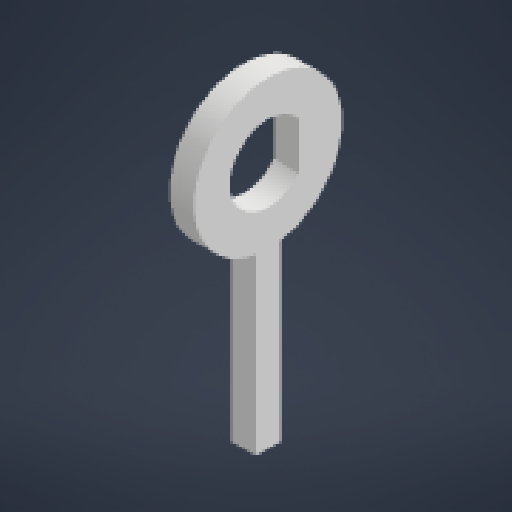
# Autodesk Inventor part: tarcza krańcówek
Saved by Autodesk Inventor 2026.1 (Build 301233020, 233B)
## iProperties
Created: 2026-03-17
Part Number: tarcza krańcówek
Material: Generic
Document SubType Name: Modeling
Designer: Jan
Density: 1 g/cm^3
Appearance: Default
Author: Jan
Autodesk Inventor part; units mm, degrees
ref_plane "YZ Plane" through (0, 0, 0) normal (1, 0, 0) x (0, 1, 0)
ref_plane "XZ Plane" through (0, 0, 0) normal (0, 1, 0) x (-1, 0, 0)
ref_plane "XY Plane" through (0, 0, 0) normal (0, 0, 1) x (1, 0, 0)
sketch "Sketch1" plane through (0, 0, 0) normal (1, 0, 0) x (0, 1, 0)
  arc A0 (1.9313, -2.4249) -> (-1.9054, -2.4453) centre (0, 0) ccw
  circle A1 centre (0, 0) radius 6
  line L0 (-3.1, 0) -> (-3.1, 2) construction
  line L1 (-1.9054, -2.4453) -> (1.9313, -2.4249)
  line L2 (0, 1) -> (-20, 1)
  line L3 (-20, 1) -> (-20, -1)
  line L4 (-20, -1) -> (0, -1)
  line L5 (0, -1) -> (0, 1)
  point P0 (-5.9161, -1)
  point P1 (-5.9161, 1)
  dimension "d0" = 6.2
  dimension "d1" = 12
  dimension "d2" = 2
  dimension "d5" = 1
  dimension "d6" = 2
  dimension "d7" = 20
  constraints: 12 end point, 3 point on circle, 2 centre point, 2 coincident, 2 parallel, 1 horizontal, 1 perpendicular, 1 tangent, 1 vertical
  measures "d0" diameter of A0
  measures "d1" diameter of A1
  measures "d2" distance of L0.start L0.end
  measures "d5" distance from line of L2 A0.centre
  measures "d6" distance of L4.end L2.start
  measures "d7" distance between parallel lines of L5 L3
extrude "Extrusion1" add sketch "Sketch1" along normal blind 2 contours A0 L2 A1 L4 L1 | A0 L4 A1 L2 | A1 L4 L3 L2
equation "\"d6\" = 2 * d5"
body "Solid1"
